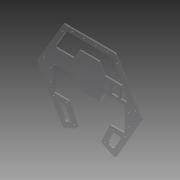
# Autodesk Inventor part: Top Plat
Saved by Autodesk Inventor 2015 (Build 190159000, 159)
## iProperties
Created: 2016-10-14
Part Number: Top Plat
Material: Polycarbonate, Clear
Document SubType Name: Modeling
Designer: James Yelland
Density: 1.2 g/cm^3
Appearance: Polycarbonate - Clear
Author: James Yelland
Autodesk Inventor part; units mm, degrees
ref_plane "YZ Plane" through (0, 0, 0) normal (1, 0, 0) x (0, 1, 0)
ref_plane "XZ Plane" through (0, 0, 0) normal (0, 1, 0) x (-1, 0, 0)
ref_plane "XY Plane" through (0, 0, 0) normal (0, 0, 1) x (1, 0, 0)
sketch "Sketch1" plane through (0, 0, 0) normal (0, 1, 0) x (-1, 0, 0)
  circle A0 centre (-30.6147, -73.9104) radius 1.6
  circle A1 centre (-30.6147, -73.9104) radius 1.6
  line L0 (-54.8095, -86.9325) -> (-103.5566, -2.5)
  line L1 (-103.5566, 2.5) -> (-53.9434, 88.4327)
  line L2 (-49.6132, 90.9327) -> (49.6132, 90.9327)
  line L3 (53.9434, 88.4327) -> (103.5566, 2.5)
  arc A2 (-54.8095, -86.9325) -> (-48.3297, -88.9468) centre (-50.4794, -84.4325) ccw
  arc A3 (-103.5566, 2.5) -> (-103.5566, -2.5) centre (-99.2265, 0) ccw
  arc A4 (-49.6132, 90.9327) -> (-53.9434, 88.4327) centre (-49.6132, 85.9327) ccw
  arc A5 (53.9434, 88.4327) -> (49.6132, 90.9327) centre (49.6132, 85.9327) ccw
  arc A6 (103.5566, -2.5) -> (103.5566, 2.5) centre (99.2265, 0) ccw
  arc A7 (-43.8396, 80.9325) -> (-48.1698, 78.4325) centre (-43.8396, 75.9325) ccw
  circle A8 centre (-30.6147, -73.9104) radius 1.6
  circle A9 centre (-30.6147, -73.9104) radius 1.6
  arc A10 (-50.7681, -73.9321) -> (-44.2883, -75.9464) centre (-46.4379, -71.4321) ccw
  arc A11 (48.1698, 78.4325) -> (43.8396, 80.9325) centre (43.8396, 75.9325) ccw
  circle A12 centre (35.5991, 85.9437) radius 1.6
  circle A13 centre (-35.5945, 85.9327) radius 1.6
  circle A14 centre (92.2171, 12.1406) radius 1.6
  circle A15 centre (-92.2171, 12.1406) radius 1.6
  line L4 (-18.2679, -8.3495) -> (18.2679, -8.3495)
  line L5 (-62.8455, -53.0133) -> (-50.7681, -73.9321)
  line L6 (59.1367, 11.2915) -> (33.0718, 11.2915)
  line L7 (59.1367, 11.2915) -> (68.2171, 11.2915)
  line L8 (-62.25, 35.5415) -> (-62.25, 17.0415)
  line L9 (-62.25, 17.0415) -> (-74.75, 17.0415)
  line L10 (-74.75, 17.0415) -> (-74.75, 35.5415)
  line L11 (-74.75, 35.5415) -> (-62.25, 35.5415)
  line L12 (-62.25, 35.5415) -> (-74.75, 17.0415) construction
  line L13 (-62.25, 17.0415) -> (-74.75, 35.5415) construction
  line L14 (30.4737, 9.7915) -> (20.866, -6.8495)
  line L15 (-30.4737, 9.7915) -> (-20.866, -6.8495)
  arc A16 (33.0718, 11.2915) -> (30.4737, 9.7915) centre (33.0718, 8.2915) ccw
  arc A17 (64.417, 41.2915) -> (67.0151, 45.7915) centre (64.417, 44.2915) ccw
  arc A18 (30.4737, 42.7915) -> (33.0718, 41.2915) centre (33.0718, 44.2915) ccw
  arc A19 (18.2679, -8.3495) -> (20.866, -6.8495) centre (18.2679, -5.3495) ccw
  arc A20 (-20.866, -6.8495) -> (-18.2679, -8.3495) centre (-18.2679, -5.3495) ccw
  arc A21 (-30.4737, 9.7915) -> (-33.0718, 11.2915) centre (-33.0718, 8.2915) ccw
  arc A22 (-33.0718, 41.2915) -> (-30.4737, 42.7915) centre (-33.0718, 44.2915) ccw
  arc A23 (-18.2679, 60.9325) -> (-20.866, 59.4325) centre (-18.2679, 57.9325) ccw
  arc A24 (20.866, 59.4325) -> (18.2679, 60.9325) centre (18.2679, 57.9325) ccw
  arc A25 (-67.0151, 45.7915) -> (-64.417, 41.2915) centre (-64.417, 44.2915) ccw
  line L16 (43.8396, 80.9325) -> (-43.8396, 80.9325)
  line L17 (-48.1698, 78.4325) -> (-67.0151, 45.7915)
  line L18 (-64.417, 41.2915) -> (-33.0718, 41.2915)
  line L19 (-30.4737, 42.7915) -> (-20.866, 59.4325)
  line L20 (-18.2679, 60.9325) -> (18.2679, 60.9325)
  line L21 (20.866, 59.4325) -> (30.4737, 42.7915)
  line L22 (33.0718, 41.2915) -> (64.417, 41.2915)
  line L23 (67.0151, 45.7915) -> (48.1698, 78.4325)
  line L24 (-56.75, 35.5415) -> (-56.75, 17.0415)
  line L25 (-56.75, 17.0415) -> (-44.25, 17.0415)
  line L26 (-44.25, 17.0415) -> (-44.25, 35.5415)
  line L27 (-44.25, 35.5415) -> (-56.75, 35.5415)
  line L28 (-56.75, 35.5415) -> (-44.25, 17.0415) construction
  line L29 (-56.75, 17.0415) -> (-44.25, 35.5415) construction
  circle A26 centre (-55.4009, 75.9081) radius 1.6
  circle A27 centre (55.3868, 75.9325) radius 1.6
  line L30 (-17.5, 81.9327) -> (17.5, 81.9327)
  line L31 (17.5, 81.9327) -> (17.5, 89.9327)
  line L32 (17.5, 89.9327) -> (-17.5, 89.9327)
  line L33 (-17.5, 89.9327) -> (-17.5, 81.9327)
  circle A28 centre (-12, 85.9327) radius 1.45
  circle A29 centre (12, 85.9327) radius 1.45
  line L34 (0, 90.9327) -> (0, 89.9327)
  line L35 (0, 89.9327) -> (0, 81.9327)
  line L36 (-74.2171, -27.8594) -> (-74.2171, 7.1406)
  line L37 (-74.2171, 7.1406) -> (-82.2171, 7.1406)
  line L38 (-82.2171, 7.1406) -> (-82.2171, -27.8594)
  line L39 (-82.2171, -27.8594) -> (-74.2171, -27.8594)
  circle A30 centre (-78.2171, -22.3594) radius 1.45
  circle A31 centre (-78.2171, 1.6406) radius 1.45
  line L40 (-82.2171, -10.3594) -> (-74.2171, -10.3594)
  line L41 (82.2171, -27.8594) -> (82.2171, 7.1406)
  line L42 (82.2171, 7.1406) -> (74.2171, 7.1406)
  line L43 (74.2171, 7.1406) -> (74.2171, -27.8594)
  line L44 (74.2171, -27.8594) -> (82.2171, -27.8594)
  circle A32 centre (78.2171, -22.3594) radius 1.45
  circle A33 centre (78.2171, 1.6406) radius 1.45
  line L45 (74.2171, -10.3594) -> (82.2171, -10.3594)
  line L46 (-77.2134, -47.5133) -> (-42.2134, -47.5133)
  line L47 (-42.2134, -47.5133) -> (-42.2134, -39.5133)
  line L48 (-42.2134, -39.5133) -> (-77.2134, -39.5133)
  line L49 (-77.2134, -39.5133) -> (-77.2134, -47.5133)
  circle A34 centre (-71.7134, -43.5133) radius 1.45
  circle A35 centre (-47.7134, -43.5133) radius 1.45
  line L50 (92.2171, 12.1406) -> (97.2171, 12.1406) construction
  line L51 (-92.2171, 12.1406) -> (-87.2171, 12.1406) construction
  arc A36 (71.2171, 8.2915) -> (68.2171, 11.2915) centre (68.2171, 8.2915) ccw
  line L52 (-33.0718, 11.2915) -> (-68.2171, 11.2915)
  line L53 (-68.2171, -38.5133) -> (-43.8241, -38.5133)
  line L54 (-71.2171, -38.5133) -> (-41.9298, -38.5133) construction
  line L55 (-71.2171, 8.2915) -> (-71.2171, -35.5133)
  arc A37 (-68.2171, 11.2915) -> (-71.2171, 8.2915) centre (-68.2171, 8.2915) ccw
  line L56 (-38.1553, -69.7034) -> (-47.4299, -50.2237)
  line L57 (-39.5741, -73.7016) -> (-44.2883, -75.9464)
  line L58 (-50.1385, -48.5133) -> (-60.2475, -48.5133)
  arc A38 (-41.1155, -40.2237) -> (-43.8241, -38.5133) centre (-43.8241, -41.5133) ccw
  arc A39 (-47.4299, -50.2237) -> (-50.1385, -48.5133) centre (-50.1385, -51.5133) ccw
  arc A40 (-60.2475, -48.5133) -> (-62.8455, -53.0133) centre (-60.2475, -51.5133) ccw
  arc A41 (-39.5741, -73.7016) -> (-38.1553, -69.7034) centre (-40.8639, -70.993) ccw
  arc A42 (-71.2171, -35.5133) -> (-68.2171, -38.5133) centre (-68.2171, -35.5133) ccw
  line L59 (-24.8278, -74.4329) -> (-41.1155, -40.2237)
  line L60 (-26.2467, -78.4311) -> (-48.3297, -88.9468)
  arc A43 (-26.2467, -78.4311) -> (-24.8278, -74.4329) centre (-27.5365, -75.7225) ccw
  circle A44 centre (30.6147, -73.9104) radius 1.6
  circle A45 centre (30.6147, -73.9104) radius 1.6
  line L61 (54.8095, -86.9325) -> (103.5566, -2.5)
  arc A46 (48.3297, -88.9468) -> (54.8095, -86.9325) centre (50.4794, -84.4325) ccw
  circle A47 centre (30.6147, -73.9104) radius 1.6
  circle A48 centre (30.6147, -73.9104) radius 1.6
  arc A49 (44.2883, -75.9464) -> (50.7681, -73.9321) centre (46.4379, -71.4321) ccw
  line L62 (62.8455, -53.0133) -> (50.7681, -73.9321)
  circle A50 centre (47.7134, -43.5133) radius 1.45
  line L63 (42.2134, -47.5133) -> (42.2134, -39.5133)
  line L64 (77.2134, -47.5133) -> (42.2134, -47.5133)
  line L65 (42.2134, -39.5133) -> (77.2134, -39.5133)
  circle A51 centre (71.7134, -43.5133) radius 1.45
  line L66 (77.2134, -39.5133) -> (77.2134, -47.5133)
  line L67 (68.2171, -38.5133) -> (43.8241, -38.5133)
  line L68 (71.2171, -38.5133) -> (41.9298, -38.5133) construction
  line L69 (71.2171, 8.2915) -> (71.2171, -35.5133)
  line L70 (38.1553, -69.7034) -> (47.4299, -50.2237)
  line L71 (39.5741, -73.7016) -> (44.2883, -75.9464)
  line L72 (50.1385, -48.5133) -> (60.2475, -48.5133)
  arc A52 (43.8241, -38.5133) -> (41.1155, -40.2237) centre (43.8241, -41.5133) ccw
  arc A53 (50.1385, -48.5133) -> (47.4299, -50.2237) centre (50.1385, -51.5133) ccw
  arc A54 (62.8455, -53.0133) -> (60.2475, -48.5133) centre (60.2475, -51.5133) ccw
  arc A55 (38.1553, -69.7034) -> (39.5741, -73.7016) centre (40.8639, -70.993) ccw
  arc A56 (68.2171, -38.5133) -> (71.2171, -35.5133) centre (68.2171, -35.5133) ccw
  line L73 (24.8278, -74.4329) -> (41.1155, -40.2237)
  line L74 (26.2467, -78.4311) -> (48.3297, -88.9468)
  arc A57 (24.8278, -74.4329) -> (26.2467, -78.4311) centre (27.5365, -75.7225) ccw
  point P0 (105, 0)
  point P1 (-105, 0)
  point P2 (-52.5, 90.9327)
  point P3 (52.5, 90.9327)
  point P4 (-93.4528, 0)
  point P5 (-46.7264, 80.9325)
  point P6 (46.7264, 80.9325)
  point P7 (-5, -80.9325)
  point P8 (5, -80.9325)
  point P9 (92.0094, -2.5)
  point P10 (69.6132, 41.2915)
  point P11 (86.9337, 11.2915)
  point P12 (-69.6132, 41.2915)
  point P13 (85.2016, 11.2915)
  point P14 (0, -8.3495)
  point P15 (-59.7134, -39.5133)
  point P16 (-59.7134, -47.5133)
  point P17 (-70.9879, -38.9104)
  point P18 (-62.905, -52.9104)
  point P19 (59.7134, -47.5133)
  point P20 (59.7134, -39.5133)
  point P21 (70.9879, -38.9104)
  point P22 (62.905, -52.9104)
  dimension "d234" = 18.5
  dimension "d249" = 35
  dimension "d250" = 8
  dimension "d252" = 2.9
  dimension "d254" = 2.9
  dimension "d255" = 1
  dimension "d256" = 35
  dimension "d257" = 8
  dimension "d258" = 2.9
  dimension "d259" = 2.9
  dimension "d261" = 35
  dimension "d262" = 8
  dimension "d263" = 2.9
  dimension "d264" = 2.9
  dimension "d266" = 35
  dimension "d267" = 8
  dimension "d268" = 2.9
  dimension "d269" = 2.9
  dimension "d297" = 3
  dimension "d299" = 3
  dimension "d300" = 3
  dimension "d303" = 3
  constraints: 150 end point, 69 point on circle, 58 centre point, 43 symmetric about line, 20 point on line, 11 tangent, 10 midpoint, 4 coincident, 3 equal radius, 14 other
  measures "d234" distance of L8.start L8.end
  measures "d249" distance of L30.start L30.end
  measures "d250" distance of L31.end L30.end
  measures "d252" diameter of A28
  measures "d254" diameter of A29
  measures "d255" distance of L34.start L34.end
  measures "d256" distance of L36.start L37.start
  measures "d257" distance of L37.end L37.start
  measures "d258" diameter of A30
  measures "d259" diameter of A31
  measures "d261" distance of L41.start L42.start
  measures "d262" distance of L42.end L42.start
  measures "d263" diameter of A32
  measures "d264" diameter of A33
  measures "d266" distance of L46.start L47.start
  measures "d267" distance of L47.end L47.start
  measures "d268" diameter of A34
  measures "d269" diameter of A35
  measures "d297" radius of A37
  measures "d299" radius of A38
  measures "d300" radius of A39
  measures "d303" radius of A43
extrude "Extrusion2" add sketch "Sketch1" along normal blind 3 contours L0 A3 L1 A4 L2 A5 L3 A6 L61 A46 L74 A57 L73 A52 L67 A56 L69 A36 L7 L6 A16 L14 A19 L4 A20 L15 A21 L52 A37 L55 A42 L53 A38 L59 A43 L60 A2 | L33 L32 L35 L30 | L35 L32 L31 L30 | L39 L38 L40 L36 | L40 L38 L37 L36 | L44 L43 L45 L41 | L45 L43 L42 L41 | L49 L48 L47 L46 | L63 L65 L66 L64
sketch "Sketch2" plane through (0, 3, 0) normal (0, 1, 0) x (1, 0, 0)
  line L0 (-23.051, -6.2915) -> (23.0507, -6.2915) construction
  line L1 (23.0507, -6.2915) -> (23.0507, -46.2915) construction
  line L2 (23.0507, -46.2915) -> (-23.051, -46.2915) construction
  line L3 (-23.051, -46.2915) -> (-23.051, -6.2915) construction
  line L4 (18.2679, 8.3495) -> (-18.2679, 8.3495) projected
  line L5 (-18.2679, -60.9325) -> (18.2679, -60.9325) projected
  line L6 (0, 8.3495) -> (0, -6.2915)
  point P0 (0, 0)
  dimension "d323" = 23.051
  constraints: 2 end point, 1 midpoint, 1 perpendicular, 1 point on line, 2 other
  measures "d323" distance between parallel lines of L3 L6
decal "Decal1"
body "Solid2"
